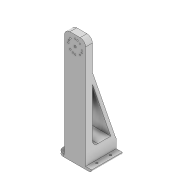
# Autodesk Inventor part: Vertical_Stereo_1
Saved by Autodesk Inventor 2022 (Build 260153000, 153)
## iProperties
Created: 2023-01-11
Part Number: Vertical_Stereo_1
Material: Generic
Document SubType Name: Modeling
Designer: MVeszpremi
Density: 1 g/cm^3
Appearance: Default
Author: MVeszpremi
Autodesk Inventor part; units mm, degrees
ref_plane "YZ Plane" through (0, 0, 0) normal (1, 0, 0) x (0, 1, 0)
ref_plane "XZ Plane" through (0, 0, 0) normal (0, 1, 0) x (-1, 0, 0)
ref_plane "XY Plane" through (0, 0, 0) normal (0, 0, 1) x (1, 0, 0)
sketch "Sketch1" plane through (0, 0, 0) normal (0, 1, 0) x (-1, 0, 0)
  line L0 (-10, -10) -> (10, -10)
  line L1 (10, -10) -> (10, 10)
  line L2 (10, 10) -> (-10, 10)
  line L3 (-10, 10) -> (-10, -10)
  line L4 (-10, -10) -> (10, 10) construction
  line L5 (10, -10) -> (-10, 10) construction
  line L6 (10, 10) -> (30, 10)
  line L7 (30, 10) -> (30, -10)
  line L8 (30, -10) -> (10, -10)
  line L9 (10, -10) -> (10, 10)
  circle A0 centre (30, 10) radius 1.5
  circle A1 centre (30, -10) radius 1.5
  circle A2 centre (10, -10) radius 1.5
  circle A3 centre (10, 10) radius 1.5
  circle A4 centre (-10, 10) radius 1.5
  circle A5 centre (-10, -10) radius 1.5
  line L10 (-15, 22.5) -> (35, 22.5)
  line L11 (35, 22.5) -> (35, -22.5)
  line L12 (35, -22.5) -> (-15, -22.5)
  line L13 (-15, -22.5) -> (-15, 22.5)
  line L14 (-15, 22.5) -> (35, -22.5) construction
  line L15 (35, 22.5) -> (-15, -22.5) construction
  point P0 (0, 0)
  point P1 (10, 0)
  dimension "d0" = 20
  dimension "d1" = 20
  dimension "d2" = 20
  dimension "d3" = 20
  dimension "d4" = 3
  dimension "d5" = 3
  dimension "d6" = 3
  dimension "d7" = 3
  dimension "d8" = 3
  dimension "d9" = 3
  dimension "d10" = 5
  dimension "d11" = 12.5
  constraints: 32 end point, 6 centre point, 6 parallel, 5 coincident, 5 midpoint, 3 horizontal, 3 perpendicular, 1 point on line
  measures "d0" distance of L1.end L2.end
  measures "d1" distance of L0.end L1.end
  measures "d2" distance of L1.end L6.end
  measures "d3" distance of L6.end L7.end
  measures "d4" diameter of A0
  measures "d5" diameter of A1
  measures "d6" diameter of A2
  measures "d7" diameter of A3
  measures "d8" diameter of A5
  measures "d9" diameter of A4
  measures "d10" distance between parallel lines of L11 L7
  measures "d11" distance between parallel lines of L6 L10
extrude "Extrusion1" add sketch "Sketch1" along normal blind 4 contours A5 L3 A4 L2 A3 L1 A2 L0 | L1 A3 L6 A0 L7 A1 L8 A2 | L10 L11 L12 L13
fillet "Fillet1" radius 4 1 edges at (15, 0, 0)
sketch "Sketch2" plane through (0, 4, 0) normal (0, 1, 0) x (1, 0, 0)
  line L0 (-35, -22.5) -> (15, -22.5) projected
  line L1 (15, 22.5) -> (-35, 22.5) projected
  line L2 (-25, -22.5) -> (6, -22.5)
  line L3 (6, -22.5) -> (6, 22.5)
  line L4 (6, 22.5) -> (-25, 22.5)
  line L5 (-25, 22.5) -> (-25, -22.5)
  line L6 (-35, 22.5) -> (-35, -22.5) projected
  line L7 (15, -22.5) -> (15, 22.5) projected
  circle A0 centre (-10, -10) radius 1.5 projected
  circle A1 centre (-10, -10) radius 4.5
  circle A2 centre (-10, 10) radius 1.5 projected
  circle A3 centre (-10, 10) radius 4.5
  point P0 (0, 0)
  point P1 (-6.25, -15)
  point P2 (-13.75, -15)
  point P3 (-13.75, 15)
  point P4 (-6.25, 15)
  dimension "d15" = 10
  dimension "d16" = 9
  dimension "d17" = 9
  dimension "d18" = 9
  constraints: 8 end point, 2 centre point, 2 coincident, 2 parallel, 2 point on line, 1 horizontal, 1 perpendicular
  measures "d15" distance between parallel lines of L6 L5
  measures "d16" distance between parallel lines of L7 L3
  measures "d17" diameter of A1
  measures "d18" diameter of A3
extrude "Extrusion2" cut sketch "Sketch2" against normal blind 4 contours A0 | A1 | A3
extrude "Extrusion3" add sketch "Sketch2" along normal blind 160 contours L5 L1 L3 L0 | A0 | A1 | A2 | A3
fillet "Fillet2" radius 8 2 edges at (-35, 2, 22.5) (-35, 2, -22.5)
sketch "Sketch3" plane through (-25, 164, 22.5) normal (0, 0, 1) x (1, 0, 0)
  line L0 (31, 0) -> (0, 0) projected
  circle A0 centre (15.8021, -15) radius 10
  circle A1 centre (15.8021, -5) radius 1
  circle A2 centre (19.2223, -5.6031) radius 1
  circle A3 centre (22.8732, -7.9289) radius 1
  line L1 (15.8021, -15) -> (19.2223, -5.6031)
  line L2 (15.8021, -15) -> (22.8732, -7.9289)
  circle A4 centre (5.8021, -15) radius 1
  circle A5 centre (15.8021, -25) radius 1
  circle A6 centre (25.8021, -15) radius 1
  circle A7 centre (6.4052, -11.5798) radius 1
  circle A8 centre (12.3819, -24.3969) radius 1
  circle A9 centre (25.199, -18.4202) radius 1
  circle A10 centre (8.731, -7.9289) radius 1
  circle A11 centre (8.731, -22.0711) radius 1
  circle A12 centre (22.8732, -22.0711) radius 1
  line L3 (15.8021, -15) -> (15.8021, 0)
  point P0 (25, -164)
  dimension "d24" = 20
  dimension "d26" = 2
  dimension "d27" = 2
  dimension "d30" = 2
  dimension "d33" = 360
  dimension "d37" = 360
  dimension "d41" = 360
  dimension "d54" = 15
  dimension "d55" = 45
  dimension "d56" = 20
  constraints: 13 centre point, 6 end point, 3 point on circle, 2 point on line, 1 perpendicular, 27 other
  measures "d24" diameter of A0
  measures "d26" diameter of A1
  measures "d27" diameter of A2
  measures "d30" diameter of A3
  measures "d54" distance of L1.start L3.end
  measures "d55" angle of L3 L2
  measures "d56" angle of L3 L1
extrude "Extrusion4" cut sketch "Sketch3" against normal blind 100 contours A0 A6 | A0 A6 | A3 L2 A0 | A0 A3 | A9 A0 | A0 A9 | L2 A3 A0 | A12 A0 | A0 A12 | A2 L1 A0 | A0 A2 | A2 A0 L1 | L3 A0 A1 | A1 A0 L3 | A1 L3 A0 | A0 L3 A1 | A5 A0 | A0 A5 | A10 A0 | A0 A10 | A8 A0 | A0 A8 | A7 A0 | A0 A7 | A11 A0 | A0 A11 | A4 A0 | A0 A4
sketch "Sketch4" plane through (0, 164, 0) normal (0, 1, 0) x (1, 0, 0)
  line L0 (-25, 22.5) -> (-25, -22.5) projected
  line L1 (6, 22.5) -> (-25, 22.5) projected
  line L2 (-25, -12.5) -> (6, -12.5)
  line L3 (6, -12.5) -> (6, 22.5)
  line L4 (6, 22.5) -> (-25, 22.5)
  line L5 (-25, 22.5) -> (-25, -12.5)
  line L6 (-25, -22.5) -> (6, -22.5) projected
  point P0 (0, 0)
  dimension "d45" = 10
  constraints: 8 end point, 2 parallel, 1 horizontal, 1 perpendicular, 1 point on line
  measures "d45" distance between parallel lines of L6 L2
extrude "Extrusion5" cut sketch "Sketch4" against normal blind 140
fillet "Fillet3" radius 8 1 edges at (-9.5, 24, 12.5)
fillet "Fillet4" radius 8 2 edges at (-25, 164, 17.5) (6, 164, 17.5)
fillet "Fillet5" radius 8 1 edges at (-9.5, 24, -22.5)
sketch "Sketch5" plane through (6, 4, 22.5) normal (1, 0, 0) x (0, 0, -1)
  line L0 (10, 28) -> (10, 152) projected
  line L1 (18, 20) -> (37, 20) projected
  line L2 (10, 99.4385) -> (37, 20)
  arc A0 (45, 12) -> (37, 20) centre (37, 12) ccw projected
  line L3 (10, 114.9758) -> (45, 12)
  arc A1 (45, 12) -> (37, 20) centre (37, 12) ccw projected
  line L4 (37, 20) -> (18, 20) projected
  arc A2 (10, 28) -> (18, 20) centre (18, 28) ccw projected
  line L5 (10, 28) -> (10, 152) projected
  line L6 (0, 152) -> (10, 152) projected
  line L7 (0, 0) -> (0, 152) projected
  line L8 (45, 0) -> (0, 0) projected
  line L9 (45, 0) -> (45, 12) projected
  point P0 (22.5, -4)
  point P1 (43.3431, 16.875)
  dimension "d51" = 5
  constraints: 4 end point, 2 point on line, 1 parallel
  measures "d51" distance between parallel lines of L3 L2
extrude "Extrusion6" add sketch "Sketch5" against normal up to surface (31 mm away) contours L0 L3 A0 L2
sketch "Sketch6" plane through (6, 4, 22.5) normal (0, 0, 1) x (1, 0, 0)
  circle A0 centre (-15.1979, 155) radius 1 projected
  circle A1 centre (-15.1979, 135) radius 1 projected
  line L0 (-15.1979, 155) -> (-15.1979, 135)
  circle A2 centre (-15.1979, 145) radius 1.5
  point P0 (-6, -4)
  dimension "d57" = 3
  constraints: 2 end point, 1 centre point, 1 midpoint, 1 vertical
  measures "d57" diameter of A2
extrude "Extrusion7" cut sketch "Sketch6" against normal blind 20 contours A2 L0 | L0 A2
body "Solid1"
